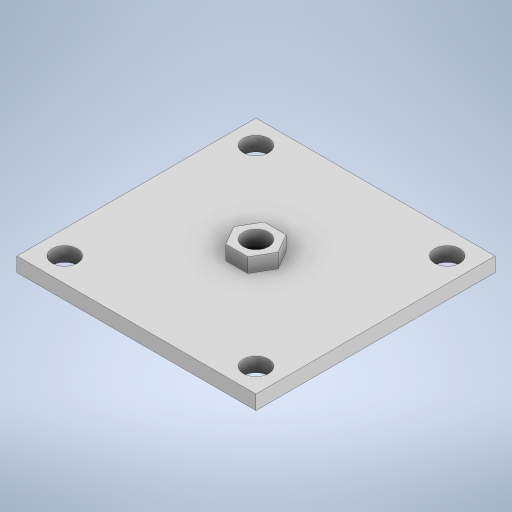
# Autodesk Inventor part: BoxLed
Saved by Autodesk Inventor 2023 (Build 270158000, 158)
## iProperties
Created: 2023-12-17
Part Number: BoxLed
Material: Generic
Document SubType Name: Modeling
Designer: Mustapha
Density: 1 g/cm^3
Appearance: Default
Author: Mustapha
Autodesk Inventor part; units mm, degrees
ref_plane "YZ Plane" through (0, 0, 0) normal (1, 0, 0) x (0, 1, 0)
ref_plane "XZ Plane" through (0, 0, 0) normal (0, 1, 0) x (-1, 0, 0)
ref_plane "XY Plane" through (0, 0, 0) normal (0, 0, 1) x (1, 0, 0)
sketch "Sketch1" plane through (0, 0, 0) normal (0, 1, 0) x (-1, 0, 0)
  line L0 (0, 0) -> (50, 0)
  line L1 (50, 0) -> (50, -50)
  line L2 (50, -50) -> (0, -50)
  line L3 (0, -50) -> (0, 0)
  circle A0 centre (45, -5) radius 2.65
  line L4 (50, -25) -> (0, -25)
  line L5 (25, -50) -> (25, 0)
  circle A1 centre (45, -45) radius 2.65
  circle A2 centre (5, -5) radius 2.65
  circle A3 centre (5, -45) radius 2.65
  dimension "d0" = 50
  dimension "d1" = 50
  dimension "d2" = 5
  dimension "d3" = 5
  dimension "d4" = 5.3
  constraints: 12 end point, 4 centre point, 4 midpoint, 3 symmetric about line, 2 parallel, 1 horizontal, 1 perpendicular, 3 other
  measures "d0" distance between parallel lines of L2 L0
  measures "d1" distance of L1.end L2.end
  measures "d2" distance from line of L1 A0.centre
  measures "d3" distance from line of L0 A0.centre
  measures "d4" diameter of A0
extrude "Extrusion1" add sketch "Sketch1" along normal blind 3
sketch "Sketch2" plane through (0, 3, 0) normal (0, 1, 0) x (1, 0, 0)
  line L0 (-20.3812, 25) -> (-22.6906, 21)
  line L1 (-22.6906, 21) -> (-27.3094, 21)
  line L2 (-27.3094, 21) -> (-29.6188, 25)
  line L3 (-29.6188, 25) -> (-27.3094, 29)
  line L4 (-27.3094, 29) -> (-22.6906, 29)
  line L5 (-22.6906, 29) -> (-20.3812, 25)
  line L6 (0, 50) -> (-50, 50) projected
  line L7 (0, 0) -> (0, 50) projected
  point P0 (-25, 25)
  point P1 (-25, 21)
  dimension "d7" = 8
  dimension "d8" = 25
  dimension "d9" = 25
  constraints: 12 end point, 1 midpoint, 1 parallel, 13 other
  measures "d7" distance from line of point (-25, 21) L4
  measures "d8" distance from line of L6 point (-25, 25)
  measures "d9" distance from line of L7 point (-25, 25)
extrude "Extrusion2" add sketch "Sketch2" along normal blind 3
sketch "Sketch3" plane through (0, 6, 0) normal (0, 1, 0) x (1, 0, 0)
  circle A0 centre (-25, 25) radius 2.65
  line L0 (0, 50) -> (-50, 50) projected
  line L1 (0, 0) -> (0, 50) projected
  dimension "d13" = 5.3
  dimension "d14" = 25
  dimension "d15" = 25
  constraints: 1 centre point
  measures "d13" diameter of A0
  measures "d14" distance from line of L0 A0.centre
  measures "d15" distance from line of L1 A0.centre
extrude "Extrusion3" cut sketch "Sketch3" against normal blind 10
body "Solid1"
